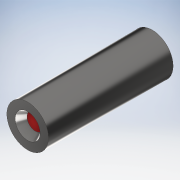
# Autodesk Inventor part: VLM-650-03-LPT
Saved by Autodesk Inventor 2018 (Build 220112000, 112)
## iProperties
Created: 2018-01-13
Part Number: VLM-650-03-LPT
Material: Generic
Document SubType Name: Modeling
Designer: Moochster
Density: 1 g/cm^3
Appearance: Semi-Polished
Mass: 0.79549 g
Surface Area: 5.47209 cm^2
Volume: 0.79549 cm^3
Author: Moochster
Autodesk Inventor part; units mm, degrees
ref_plane "YZ Plane" through (0, 0, 0) normal (1, 0, 0) x (0, 1, 0)
ref_plane "XZ Plane" through (0, 0, 0) normal (0, 1, 0) x (-1, 0, 0)
ref_plane "XY Plane" through (0, 0, 0) normal (0, 0, 1) x (1, 0, 0)
sketch "Sketch1" plane through (0, 0, 0) normal (0, 0, 1) x (1, 0, 0)
  line L0 (0, 0) -> (0, 21)
  line L1 (0, 21) -> (3.5, 21)
  line L2 (3.5, 21) -> (3.5, 0)
  line L3 (3.5, 0) -> (2.1113, 0)
  line L4 (2.1113, 0) -> (1.4, 1.2923)
  line L5 (1.4, 1.2923) -> (0, 1.2923)
  dimension "d0" = 7
  dimension "d1" = 21
  constraints: 12 end point, 3 perpendicular, 1 horizontal, 1 horizontal alignment, 1 point on line, 1 vertical
  measures "d0" diameter of L2 L0
  measures "d1" distance of L1.end L2.end
revolve "Revolution1" add sketch "Sketch1" angle 360 about axis through (0, 0, 0) along (0, 1, 0)
body "Solid1"
